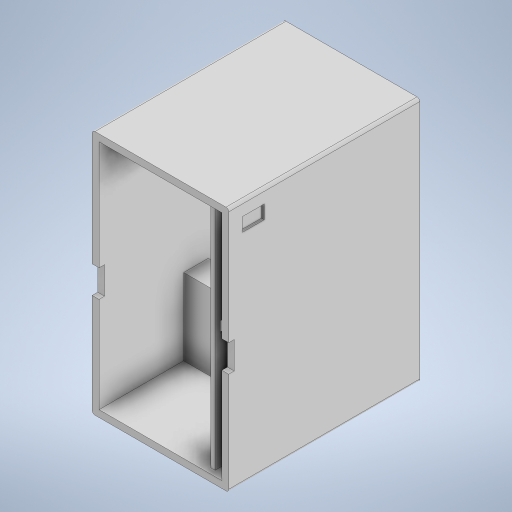
# Autodesk Inventor part: 外壳
Saved by Autodesk Inventor 2023.1 (Build 271208000, 208)
## iProperties
Created: 2023-07-19
Part Number: 外壳
Material: 常规
Document SubType Name: Modeling
Designer: Selcon
Density: 1 g/cm^3
Appearance: 默认
Author: Selcon
Autodesk Inventor part; units mm, degrees
ref_plane "YZ Plane" through (0, 0, 0) normal (1, 0, 0) x (0, 1, 0)
ref_plane "XZ Plane" through (0, 0, 0) normal (0, 1, 0) x (-1, 0, 0)
ref_plane "XY Plane" through (0, 0, 0) normal (0, 0, 1) x (1, 0, 0)
sketch "草图1" plane through (0, 0, 0) normal (0, 0, 1) x (1, 0, 0)
  line L0 (-250, 450) -> (250, 450)
  line L1 (250, 450) -> (250, -450)
  line L2 (250, -450) -> (-250, -450)
  line L3 (-250, -450) -> (-250, 450)
  line L4 (-350, 0) -> (350, 0) projected
  line L5 (0, -630) -> (0, 630) projected
  point P0 (0, 0)
  dimension "d0" = 500
  dimension "d1" = 900
  constraints: 8 end point, 2 parallel, 1 horizontal, 1 perpendicular, 2 other
  measures "d0" distance of L0.start L0.end
  measures "d1" distance of L0.end L1.end
extrude "拉伸1" add sketch "草图1" along normal mid plane 700
sketch "草图2" plane through (0, 0, 350) normal (0, 0, 1) x (1, 0, 0)
  line L0 (-225, 425) -> (225, 425)
  line L1 (225, 425) -> (225, -425)
  line L2 (225, -425) -> (-225, -425)
  line L3 (-225, -425) -> (-225, 425)
  line L4 (0, -630) -> (0, 630) projected
  line L5 (-350, 0) -> (350, 0) projected
  point P0 (0, 0)
  point P1 (225, 0)
  point P2 (0, -425)
  point P3 (-225, 0)
  point P4 (0, 425)
  dimension "d4" = 850
  dimension "d5" = 450
  constraints: 8 end point, 2 parallel, 1 horizontal, 1 perpendicular, 2 other
  measures "d4" distance of L0.end L1.end
  measures "d5" distance of L0.start L0.end
extrude "拉伸2" cut sketch "草图2" against normal blind 675
sketch "草图3" plane through (0, 0, -325) normal (0, 0, 1) x (1, 0, 0)
  line L0 (225, 425) -> (225, -425) projected
  line L1 (-225, -425) -> (165, -425)
  line L2 (165, -425) -> (165, -175)
  line L3 (165, -175) -> (-225, -175)
  line L4 (-225, -175) -> (-225, -425)
  point P0 (0, 0)
  point P1 (225, -325)
  dimension "d8" = 250
  dimension "d60" = 390
  constraints: 8 end point, 2 parallel, 1 horizontal, 1 perpendicular
  measures "d8" distance between parallel lines of L1 L3
  measures "d60" distance of L2.end L3.end
extrude "拉伸3" cut sketch "草图3" against normal through all
ref_plane "工作平面1" through (180, -425, 350) normal (-1, 0, 0) x (0, 0, 1)
sketch "草图4" plane through (225, -425, 350) normal (-1, 0, 0) x (0, 0, 1)
  line L0 (-400, 280) -> (-310, 280)
  line L1 (-310, 280) -> (-310, 0)
  line L2 (-310, 0) -> (-400, 0)
  line L3 (-400, 0) -> (-400, 280)
  line L4 (-400, -168.792) -> (-400, 811.208)
  line L5 (0, 0) -> (-675, 0) projected
  line L6 (-700, 875) -> (-700, -25) projected
  point P0 (-700, 0)
  dimension "d40" = 90
  dimension "d41" = 300
  dimension "d42" = 280
  constraints: 10 end point, 2 horizontal, 2 point on line, 1 parallel, 1 vertical
  measures "d40" distance of L0.start L0.end
  measures "d41" distance between parallel lines of L4 L6
  measures "d42" distance of L0.end L1.end
extrude "拉伸4" add sketch "草图4" along normal up to surface (450 mm away)
sketch "草图8" plane through (180, -425, 350) normal (-1, 0, 0) x (0, 0, 1)
  line L0 (-20, 0) -> (-310, 0)
  line L1 (-675, 850) -> (-20, 850)
  line L2 (-20, 850) -> (-20, 0)
  line L3 (-20, 0) -> (-675, 0)
  line L4 (-675, 0) -> (-675, 850)
  line L5 (-675, 850) -> (-675, 0) projected
  line L6 (0, 850) -> (0, 0) projected
  point P0 (-350, 425)
  point P1 (-350, 0)
  point P2 (-675, 250)
  point P3 (-275, 0)
  dimension "d33" = 850
  dimension "d117" = 20
  constraints: 10 end point, 2 parallel, 1 horizontal, 1 perpendicular, 1 point on line
  measures "d33" distance of L1.end L0.start
  measures "d117" distance between parallel lines of L6 L2
extrude "拉伸7" add sketch "草图8" along normal blind 15
sketch "草图12" plane through (225, -425, 40) normal (0, 0, 1) x (1, 0, 0)
  line L0 (0, 280) -> (-45, 280) projected
  line L1 (-45, 0) -> (0, 0) projected
  line L2 (-45, 280) -> (0, 280)
  line L3 (0, 280) -> (0, 0)
  line L4 (0, 0) -> (-45, 0)
  line L5 (-45, 0) -> (-45, 280)
  point P0 (-225, 425)
  constraints: 8 end point, 2 parallel, 1 horizontal, 1 perpendicular
extrude "拉伸8" cut sketch "草图12" against normal up to surface (90 mm away)
sketch "草图6" plane through (225, -145, -50) normal (0, 1, 0) x (1, 0, 0)
  line L0 (-270, -90) -> (-240, -90)
  line L1 (-240, -90) -> (-240, -30)
  line L2 (-240, -30) -> (-270, -30)
  line L3 (-270, -30) -> (-270, -90)
  line L4 (-60, 0) -> (-60, 300) projected
  line L5 (-450, 0) -> (-450, 300) projected
  line L6 (-255, 100.8766) -> (-255, -114.3838)
  line L7 (-60, -90) -> (-450, -90) projected
  line L8 (-60, -90) -> (-450, -90) projected
  point P0 (0, 0)
  point P1 (-60, 60)
  point P2 (-60, 275)
  point P3 (-450, 60)
  point P4 (-60, -400)
  point P5 (-255, -90)
  dimension "d14" = 60
  dimension "d15" = 30
  dimension "d35" = 390
  constraints: 10 end point, 2 midpoint, 2 parallel, 1 horizontal, 1 perpendicular, 1 vertical, 1 other
  measures "d14" distance of L0.end L1.end
  measures "d15" distance of L1.end L2.end
  measures "d35" diameter of L4 L6
extrude "拉伸5" cut sketch "草图6" against normal blind 25
sketch "草图7" plane through (225, -170, -50) normal (0, 1, 0) x (1, 0, 0)
  circle A0 centre (-255, -45) radius 6
  circle A1 centre (-255, -65) radius 6
  line L0 (-270.0194, -90) -> (-239.9806, -90)
  line L1 (-60, 0) -> (-60, 300) projected
  line L2 (-450, 0) -> (-450, 300) projected
  line L3 (-255, 158.1322) -> (-255, -68.0014)
  line L4 (-240, -90) -> (-270, -90) projected
  line L5 (-270, -90) -> (-450, -90) projected
  line L6 (-60, -90) -> (-450, -90) projected
  line L7 (-60, -90) -> (-240, -90) projected
  point P0 (-255, -90)
  point P1 (-60, 60)
  point P2 (-60, 275)
  point P3 (-450, 60)
  point P4 (-60, -400)
  point P5 (-255, -90)
  dimension "d9" = 0
  dimension "d20" = 12
  dimension "d21" = 12
  dimension "d22" = 20
  dimension "d23" = 25
  dimension "d38" = 390
  constraints: 4 end point, 3 midpoint, 3 point on line, 2 centre point, 1 vertical
  measures "d20" diameter of A0
  measures "d21" diameter of A1
  measures "d22" distance of A1.centre A0.centre
  measures "d23" distance of point (-255, -90) A1.centre
  measures "d38" diameter of L1 L3
extrude "拉伸6" cut sketch "草图7" against normal blind 25
thread "螺纹1" size "M12x1.75" class "6H" standard "ANSI Metric M Profile" full length
thread "螺纹2" size "M12x1.75" class "6H" standard "ANSI Metric M Profile" full length
fillet "圆角1" radius 10 4 edges at (-250, 450, 0) (250, 450, 0) (-250, -450, 0) (250, -450, 0)
sketch "草图14" plane through (165, -425, -350) normal (-1, 0, 0) x (0, 0, 1)
  line L0 (640, 485) -> (660, 485)
  line L1 (660, 485) -> (660, 405)
  line L2 (660, 405) -> (640, 405)
  line L3 (640, 405) -> (640, 485)
  line L4 (680, 0) -> (680, 850) projected
  line L5 (680, 0) -> (25, 0) projected
  point P0 (350, 425)
  point P1 (700, 0)
  point P2 (700, 850)
  dimension "d69" = 80
  dimension "d70" = 20
  dimension "d115" = 20
  dimension "d118" = 405
  constraints: 8 end point, 2 parallel, 1 horizontal, 1 perpendicular, 1 other
  measures "d69" distance of L0.end L1.end
  measures "d70" distance of L1.end L2.end
  measures "d118" distance between parallel lines of L5 L2
extrude "拉伸10" cut sketch "草图14" against normal blind 10
sketch "草图15" plane through (175, -425, -350) normal (-1, 0, 0) x (0, 0, 1)
  line L0 (640, 405) -> (640, 485) projected
  line L1 (660, 405) -> (640, 405) projected
  line L2 (660, 485) -> (660, 405) projected
  line L3 (640, 485) -> (660, 485) projected
  line L4 (640, 405) -> (640, 485) projected
  line L5 (640, 465) -> (660, 465)
  line L6 (660, 465) -> (660, 425)
  line L7 (660, 425) -> (640, 425)
  line L8 (640, 425) -> (640, 465)
  line L9 (565.3666, 445) -> (668.9353, 445)
  point P0 (350, 425)
  point P1 (640, 445)
  dimension "d74" = 40
  constraints: 10 end point, 3 point on line, 2 horizontal, 2 parallel, 1 midpoint, 1 perpendicular, 1 other
  measures "d74" distance between parallel lines of L7 L5
extrude "拉伸11" cut sketch "草图15" against normal up to surface (5 mm away) contours L0 L9 L2 L7 | L0 L5 L2 L9
sketch "草图17" plane through (165, -175, -325) normal (-1, 0, 0) x (0, 0, 1)
  line L0 (105, 400) -> (95, 345)
  line L1 (95, 345) -> (575, 225)
  line L2 (575, 225) -> (585, 280)
  line L3 (585, 280) -> (105, 400)
  line L4 (-25, 625) -> (675, 625) projected
  line L5 (-25, 615) -> (-25, -265) projected
  point P0 (325, 175)
  dimension "d83" = 480
  dimension "d84" = 55
  dimension "d85" = 225
  dimension "d86" = 130
  dimension "d87" = 120
  dimension "d88" = 120
  constraints: 8 end point, 2 parallel
  measures "d83" horizontal distance of L2.end L0.start
  measures "d84" vertical distance of L1.end L2.end
  measures "d85" distance from line of L4 L0.start
  measures "d86" distance from line of L5 L0.start
  measures "d87" distance from line of L5 L0.end
  measures "d88" vertical distance of L2.end L0.start
extrude "拉伸13" cut sketch "草图17" against normal up to surface (15 mm away)
sketch "草图19" plane through (250, -440, 350) normal (1, 0, 0) x (0, 0, -1)
  line L0 (50, 840) -> (130, 840)
  line L1 (130, 840) -> (130, 790)
  line L2 (130, 790) -> (50, 790)
  line L3 (50, 790) -> (50, 840)
  line L4 (700, 890) -> (0, 890) projected
  line L5 (0, 0) -> (0, 880) projected
  point P0 (350, 440)
  dimension "d93" = 80
  dimension "d94" = 50
  dimension "d95" = 50
  dimension "d96" = 50
  constraints: 8 end point, 2 parallel, 1 horizontal, 1 perpendicular
  measures "d93" distance of L0.start L0.end
  measures "d94" distance of L0.end L1.end
  measures "d95" distance from line of L4 L0.start
  measures "d96" distance from line of L5 L0.start
extrude "拉伸15" cut sketch "草图19" against normal blind 10
sketch "草图20" plane through (240, -440, 350) normal (1, 0, 0) x (0, 0, -1)
  line L0 (130, 790) -> (50, 790) projected
  line L1 (130, 840) -> (130, 790) projected
  line L2 (50, 840) -> (130, 840) projected
  line L3 (50, 790) -> (50, 840) projected
  line L4 (50, 840) -> (130, 840) projected
  line L5 (75, 840) -> (105, 840)
  line L6 (105, 840) -> (105, 835)
  line L7 (105, 835) -> (75, 835)
  line L8 (75, 835) -> (75, 840)
  line L9 (90, 871.8098) -> (90, 758.1154)
  point P0 (350, 440)
  point P1 (90, 840)
  point P2 (75, 840)
  point P3 (105, 840)
  dimension "d99" = 5
  dimension "d100" = 30
  constraints: 10 end point, 2 parallel, 2 point on line, 1 horizontal, 1 midpoint, 1 perpendicular, 1 vertical, 1 other
  measures "d99" distance of L5.end L6.end
  measures "d100" distance of L6.end L7.end
extrude "拉伸16" cut sketch "草图20" against normal up to surface (15 mm away) contours L9 L2 L6 L7 | L7 L8 L2 L9
sketch "草图23" plane through (-225, 425, 350) normal (1, 0, 0) x (0, 0, -1)
  line L0 (100, -375) -> (580, -255) projected
  line L1 (675, -200) -> (615, -200)
  line L2 (0, -850) -> (0, 0) projected
  line L3 (0, -850) -> (310, -850) projected
  line L4 (310, -850) -> (310, -570) projected
  line L5 (310, -570) -> (400, -570) projected
  line L6 (400, -570) -> (400, -850) projected
  line L7 (400, -850) -> (700, -850) projected
  line L8 (700, -600) -> (700, -850) projected
  line L9 (675, -600) -> (700, -600) projected
  line L10 (675, -600) -> (675, 0) projected
  line L11 (0, 0) -> (675, 0) projected
  line L12 (615, -200) -> (615, -400)
  line L13 (615, -400) -> (595, -400)
  line L14 (595, -400) -> (595, -165.9896)
  line L15 (595, -165.8218) -> (595, -180)
  line L16 (595, -180) -> (675, -180)
  line L17 (675, -180) -> (675, -200)
  point P0 (350, -425)
  point P1 (650, 0)
  dimension "d110" = 20
  dimension "d111" = 200
  dimension "d112" = 80
  constraints: 15 end point, 4 parallel, 3 point on line, 1 vertical
  measures "d110" distance of L12.end L13.end
  measures "d111" distance of L1.end L12.end
  measures "d112" distance of L15.end L16.end
extrude "拉伸17" add sketch "草图23" along normal up to surface (390 mm away) contours L1 L12 L13 L14 L16 L10
sketch "草图25" plane through (-250, -440, 350) normal (-1, 0, 0) x (0, 0, 1)
  line L0 (-700, 880) -> (0, 880) projected
  line L1 (-20, 465) -> (0, 465)
  line L2 (0, 465) -> (0, 365)
  line L3 (0, 365) -> (-20, 365)
  line L4 (-20, 365) -> (-20, 465)
  line L5 (0, 880) -> (0, 0) projected
  line L6 (0, 0) -> (-700, 0) projected
  point P0 (-350, 440)
  point P1 (0, 415)
  dimension "d120" = 20
  dimension "d121" = 100
  dimension "d124" = 365
  constraints: 8 end point, 2 parallel, 1 horizontal, 1 midpoint, 1 perpendicular, 1 point on line
  measures "d120" distance of L2.end L3.end
  measures "d121" distance of L3.end L1.start
  measures "d124" distance between parallel lines of L6 L3
extrude "拉伸19" cut sketch "草图25" against normal through all
